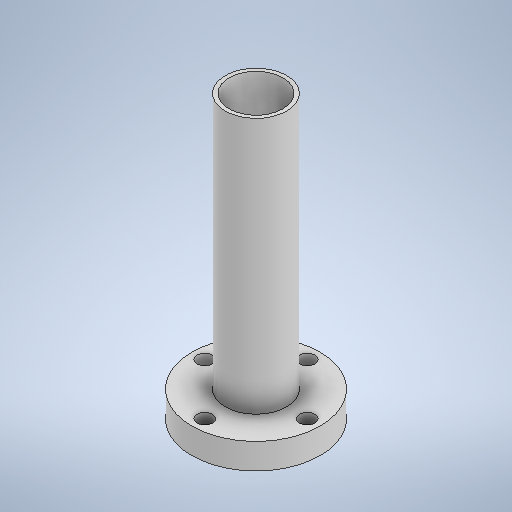
# Autodesk Inventor part: Pieza1
Saved by Autodesk Inventor 2025.2 (Build 292293000, 293)
## iProperties
Created: 2024-12-14
Part Number: Pieza1
Material: Genérico
Document SubType Name: Modeling
Designer: USER
Density: 1 g/cm^3
Appearance: Valor por defecto
Author: USER
Autodesk Inventor part; units mm, degrees
ref_plane "YZ Plane" through (0, 0, 0) normal (1, 0, 0) x (0, 1, 0)
ref_plane "XZ Plane" through (0, 0, 0) normal (0, 1, 0) x (-1, 0, 0)
ref_plane "XY Plane" through (0, 0, 0) normal (0, 0, 1) x (1, 0, 0)
sketch "Boceto1" plane through (0, 0, 0) normal (0, 1, 0) x (-1, 0, 0)
  circle A0 centre (0, 0) radius 25
  circle A1 centre (20, 0) radius 3
  circle A2 centre (0, 20) radius 3
  circle A3 centre (-20, 0) radius 3
  circle A4 centre (0, -20) radius 3
  dimension "d0" = 50
  dimension "d2" = 6
  dimension "d5" = 360
  constraints: 5 centre point, 3 coincident, 11 other
  measures "d0" diameter of A0
  measures "d2" diameter of A1
extrude "Extrusión1" add sketch "Boceto1" along normal blind 10
sketch "Boceto2" plane through (0, 10, 0) normal (0, 1, 0) x (1, 0, 0)
  circle A0 centre (0, 0) radius 12
  circle A1 centre (0, 0) radius 10.5
  dimension "d9" = 24
  dimension "d10" = 21
  constraints: 2 centre point, 2 coincident
  measures "d9" diameter of A0
  measures "d10" diameter of A1
extrude "Extrusión2" add sketch "Boceto2" along normal blind 100 contours A0 | A1
sketch "Boceto3" plane through (0, 110, 0) normal (0, 1, 0) x (1, 0, 0)
  circle A0 centre (0, 0) radius 12 projected
  constraints: 1 coincident
hole "Agujero1" at (0, 110, 0) direction (0, -1, 0) diameter 21 depth 100
